Autodesk Inventor part; units mm, degrees
(part 2 of 2)
sketch "Boceto13" plane through (0, 0, 0) normal (0, 0, -1) x (-1, 0, 0)
  circle A0 centre (-56.75, 72.0206) radius 8 projected
  line L0 (-56.75, 72.0206) -> (-80.75, 72.0206)
  line L1 (-80.75, 105.95) -> (-80.75, -105.95) projected
  line L2 (-80.75, 72.0206) -> (80.75, 72.0206)
  line L3 (80.75, -105.95) -> (80.75, 105.95) projected
  circle A1 centre (-56.75, 43.1636) radius 8 projected
  line L4 (-56.75, 43.1636) -> (-56.75, 72.0206)
  line L5 (-56.75, 43.1636) -> (-80.75, 43.1636)
  line L6 (-80.75, 43.1636) -> (80.75, 43.1636)
  line L7 (-56.75, 14.3066) -> (-56.75, 43.1636)
  line L8 (-56.75, 14.3066) -> (-80.75, 14.3066)
  line L9 (-80.75, 14.3066) -> (80.75, 14.3066)
  line L10 (-56.75, -14.5504) -> (-56.75, 14.3066)
  line L11 (-56.75, -14.5504) -> (-80.75, -14.5504)
  line L12 (-80.75, -14.5504) -> (80.75, -14.5504)
  line L13 (-56.75, -43.4074) -> (-56.75, -14.5504)
  line L14 (-56.75, -43.4074) -> (-80.75, -43.4074)
  line L15 (-80.75, -43.4074) -> (80.75, -43.4074)
  line L16 (-56.75, -72.2644) -> (-56.75, -43.4074)
  line L17 (-56.75, -98.6167) -> (-56.75, -69.7597)
  line L18 (-56.75, -72.2644) -> (-80.75, -72.2644)
  line L19 (-80.75, -72.2644) -> (80.75, -72.2644)
  line L20 (-56.75, -101.1214) -> (-56.75, -72.2644)
  line L21 (43.5, 62.1456) -> (30.5, 62.1456) projected
  line L22 (30.5, 62.1456) -> (-80.75, 62.1456)
  line L23 (30.5, 81.8956) -> (43.5, 81.8956) projected
  line L24 (30.5, 81.8956) -> (80.75, 81.8956)
  line L25 (30.5, 62.1456) -> (80.75, 62.1456)
  line L26 (30.5, 81.8956) -> (-80.75, 81.8956)
  line L27 (30.5, 33.2886) -> (-80.75, 33.2886)
  line L28 (30.5, 53.0386) -> (80.75, 53.0386)
  line L29 (30.5, 33.2886) -> (80.75, 33.2886)
  line L30 (30.5, 53.0386) -> (-80.75, 53.0386)
  line L31 (30.5, 4.4316) -> (-80.75, 4.4316)
  line L32 (30.5, 24.1816) -> (80.75, 24.1816)
  line L33 (30.5, 4.4316) -> (80.75, 4.4316)
  line L34 (30.5, 24.1816) -> (-80.75, 24.1816)
  line L35 (30.5, -24.4254) -> (-80.75, -24.4254)
  line L36 (30.5, -4.6754) -> (80.75, -4.6754)
  line L37 (30.5, -24.4254) -> (80.75, -24.4254)
  line L38 (30.5, -4.6754) -> (-80.75, -4.6754)
  line L39 (30.5, -53.2824) -> (-80.75, -53.2824)
  line L40 (30.5, -33.5324) -> (80.75, -33.5324)
  line L41 (30.5, -53.2824) -> (80.75, -53.2824)
  line L42 (30.5, -33.5324) -> (-80.75, -33.5324)
  line L43 (30.5, -82.1394) -> (-80.75, -82.1394)
  line L44 (30.5, -62.3894) -> (80.75, -62.3894)
  line L45 (30.5, -82.1394) -> (80.75, -82.1394)
  line L46 (30.5, -62.3894) -> (-80.75, -62.3894)
  line L47 (-80.6263, 81.8524) -> (-64.7122, 81.8524) construction
  line L48 (-64.7122, 81.8524) -> (-64.7122, 62.1807) construction
  line L49 (-64.7122, 62.1807) -> (-80.6263, 62.1807) construction
  line L50 (-80.6263, 62.1807) -> (-80.6263, 81.8524) construction
  line L51 (-83, 108.2) -> (83, 108.2) projected
  line L52 (0, 108.2) -> (0, -109.1206)
  line L53 (-80.6263, 52.9954) -> (-64.7122, 52.9954) construction
  line L54 (-64.7122, 52.9954) -> (-64.7122, 33.3237) construction
  line L55 (-64.7122, 33.3237) -> (-80.6263, 33.3237) construction
  line L56 (-80.6263, 33.3237) -> (-80.6263, 52.9954) construction
  line L57 (-80.6263, 24.1384) -> (-64.7122, 24.1384) construction
  line L58 (-64.7122, 24.1384) -> (-64.7122, 4.4667) construction
  line L59 (-64.7122, 4.4667) -> (-80.6263, 4.4667) construction
  line L60 (-80.6263, 4.4667) -> (-80.6263, 24.1384) construction
  line L61 (-80.6263, -4.7186) -> (-64.7122, -4.7186) construction
  line L62 (-64.7122, -4.7186) -> (-64.7122, -24.3903) construction
  line L63 (-64.7122, -24.3903) -> (-80.6263, -24.3903) construction
  line L64 (-80.6263, -24.3903) -> (-80.6263, -4.7186) construction
  line L65 (-80.6263, -33.5756) -> (-64.7122, -33.5756) construction
  line L66 (-64.7122, -33.5756) -> (-64.7122, -53.2473) construction
  line L67 (-64.7122, -53.2473) -> (-80.6263, -53.2473) construction
  line L68 (-80.6263, -53.2473) -> (-80.6263, -33.5756) construction
  line L69 (-80.6263, -62.4326) -> (-64.7122, -62.4326) construction
  line L70 (-64.7122, -62.4326) -> (-64.7122, -82.1043) construction
  line L71 (-64.7122, -82.1043) -> (-80.6263, -82.1043) construction
  line L72 (-80.6263, -82.1043) -> (-80.6263, -62.4326) construction
  line L73 (-72.6693, 72.0206) -> (-88.5883, 72.0206)
  circle A2 centre (56.75, 72.0206) radius 8 projected
  circle A3 centre (56.75, -72.2644) radius 8 projected
  line L74 (56.75, 72.0206) -> (56.75, -72.2644)
  line L75 (64.7119, 81.8524) -> (80.6261, 81.8524) construction
  line L76 (80.6261, 81.8524) -> (80.6261, 62.1807) construction
  line L77 (80.6261, 62.1807) -> (64.7119, 62.1807) construction
  line L78 (64.7119, 62.1807) -> (64.7119, 81.8524) construction
  line L79 (56.75, 43.1636) -> (56.75, 14.3066)
  line L80 (56.75, -14.5504) -> (56.75, 14.3066)
  circle A4 centre (56.75, -43.4074) radius 8 projected
  line L81 (56.75, -72.2644) -> (56.75, -43.4074)
  line L82 (56.75, -43.4074) -> (56.75, -14.5504)
  line L83 (64.7119, 33.3237) -> (64.7119, 52.9954) construction
  line L84 (64.7119, 52.9954) -> (80.6261, 52.9954) construction
  line L85 (80.6261, 52.9954) -> (80.6261, 33.3237) construction
  line L86 (80.6261, 33.3237) -> (64.7119, 33.3237) construction
  line L87 (64.7119, 4.4667) -> (64.7119, 24.1384) construction
  line L88 (64.7119, 24.1384) -> (80.6261, 24.1384) construction
  line L89 (80.6261, 24.1384) -> (80.6261, 4.4667) construction
  line L90 (80.6261, 4.4667) -> (64.7119, 4.4667) construction
  line L91 (64.7119, -24.3903) -> (64.7119, -4.7186) construction
  line L92 (64.7119, -4.7186) -> (80.6261, -4.7186) construction
  line L93 (80.6261, -4.7186) -> (80.6261, -24.3903) construction
  line L94 (80.6261, -24.3903) -> (64.7119, -24.3903) construction
  line L95 (64.7119, -53.2473) -> (64.7119, -33.5756) construction
  line L96 (64.7119, -33.5756) -> (80.6261, -33.5756) construction
  line L97 (80.6261, -33.5756) -> (80.6261, -53.2473) construction
  line L98 (80.6261, -53.2473) -> (64.7119, -53.2473) construction
  line L99 (64.7119, -82.1043) -> (64.7119, -62.4326) construction
  line L100 (64.7119, -62.4326) -> (80.6261, -62.4326) construction
  line L101 (80.6261, -62.4326) -> (80.6261, -82.1043) construction
  line L102 (80.6261, -82.1043) -> (64.7119, -82.1043) construction
  line L103 (-70.5115, 68.9591) -> (-74.5403, 68.9591)
  line L104 (-74.5403, 68.9591) -> (-74.5403, 70.0219)
  line L105 (-74.5403, 70.0219) -> (-73.2551, 70.0219)
  line L106 (-73.2551, 70.0219) -> (-73.2551, 73.2499)
  line L107 (-73.2551, 73.2499) -> (-74.5403, 73.2499)
  line L108 (-74.5403, 73.2499) -> (-74.5403, 74.2435)
  spline S0 degree 2 poles (-74.5403, 74.2435) (-74.2585, 74.2435) (-73.7, 74.3177) (-73.5319, 74.3967) knots 0 0 0 1 2 2 2
  spline S1 degree 2 poles (-73.5319, 74.3967) (-73.3391, 74.4956) (-73.1216, 74.8268) (-73.1018, 75.074) knots 0 0 0 1 2 2 2
  line L109 (-73.1018, 75.074) -> (-71.7671, 75.074)
  line L110 (-71.7671, 75.074) -> (-71.7671, 70.0219)
  line L111 (-71.7671, 70.0219) -> (-70.5115, 70.0219)
  line L112 (-70.5115, 70.0219) -> (-70.5115, 68.9591)
  line L113 (-70.2397, 40.0502) -> (-74.7232, 40.0502)
  line L114 (-74.7232, 40.0502) -> (-74.7232, 41.0438)
  spline S2 degree 2 poles (-74.7232, 41.0438) (-74.1547, 41.4986) (-73.2452, 42.2994) (-72.9041, 42.6603) knots 0 0 0 1 2 2 2
  spline S3 degree 2 poles (-72.9041, 42.6603) (-72.4542, 43.1299) (-72.0538, 43.8467) (-72.0538, 44.2224) knots 0 0 0 1 2 2 2
  spline S4 degree 2 poles (-72.0538, 44.2224) (-72.0538, 44.6475) (-72.563, 45.1023) (-73.0178, 45.1023) knots 0 0 0 1 2 2 2
  spline S5 degree 2 poles (-73.0178, 45.1023) (-73.2501, 45.1023) (-73.6653, 44.9886) (-73.8779, 44.8996) knots 0 0 0 1 2 2 2
  spline S6 degree 2 poles (-73.8779, 44.8996) (-74.0855, 44.8057) (-74.3821, 44.6079) (-74.4563, 44.5585) knots 0 0 0 1 2 2 2
  line L115 (-74.4563, 44.5585) -> (-74.5749, 44.5585)
  line L116 (-74.5749, 44.5585) -> (-74.5749, 45.8882)
  spline S7 degree 2 poles (-74.5749, 45.8882) (-74.3179, 46.0118) (-73.2205, 46.2689) (-72.7113, 46.2689) knots 0 0 0 1 2 2 2
  spline S8 degree 2 poles (-72.7113, 46.2689) (-71.6238, 46.2689) (-70.5066, 45.3) (-70.5066, 44.425) knots 0 0 0 1 2 2 2
  spline S9 degree 2 poles (-70.5066, 44.425) (-70.5066, 43.8862) (-71.0158, 42.8481) (-71.604, 42.2549) knots 0 0 0 1 2 2 2
  spline S10 degree 2 poles (-71.604, 42.2549) (-71.9748, 41.8891) (-72.6718, 41.3207) (-72.825, 41.202) knots 0 0 0 1 2 2 2
  line L117 (-72.825, 41.202) -> (-70.2397, 41.202)
  line L118 (-70.2397, 41.202) -> (-70.2397, 40.0502)
  spline S11 degree 2 poles (-70.3929, 13.1013) (-70.3929, 12.6515) (-70.7241, 11.915) (-71.0454, 11.6579) knots 0 0 0 1 2 2 2
  spline S12 degree 2 poles (-71.0454, 11.6579) (-71.3667, 11.4009) (-72.2417, 11.124) (-72.8695, 11.124) knots 0 0 0 1 2 2 2
  spline S13 degree 2 poles (-72.8695, 11.124) (-73.5813, 11.124) (-74.5996, 11.3613) (-74.9209, 11.5096) knots 0 0 0 1 2 2 2
  line L119 (-74.9209, 11.5096) -> (-74.9209, 12.8344)
  line L120 (-74.9209, 12.8344) -> (-74.7726, 12.8344)
  spline S14 degree 2 poles (-74.7726, 12.8344) (-74.4365, 12.6218) (-73.5319, 12.3055) (-73.1562, 12.3055) knots 0 0 0 1 2 2 2
  spline S15 degree 2 poles (-73.1562, 12.3055) (-72.9337, 12.3055) (-72.4147, 12.3846) (-72.2367, 12.5131) knots 0 0 0 1 2 2 2
  spline S16 degree 2 poles (-72.2367, 12.5131) (-72.0983, 12.6169) (-71.9303, 12.9184) (-71.9303, 13.1903) knots 0 0 0 1 2 2 2
  spline S17 degree 2 poles (-71.9303, 13.1903) (-71.9303, 13.4622) (-72.1675, 13.7539) (-72.3653, 13.8231) knots 0 0 0 1 2 2 2
  spline S18 degree 2 poles (-72.3653, 13.8231) (-72.563, 13.8923) (-73.1117, 13.9071) (-73.3243, 13.9071) knots 0 0 0 1 2 2 2
  line L121 (-73.3243, 13.9071) -> (-73.5863, 13.9071)
  line L122 (-73.5863, 13.9071) -> (-73.5863, 14.9798)
  line L123 (-73.5863, 14.9798) -> (-73.344, 14.9798)
  spline S19 degree 2 poles (-73.344, 14.9798) (-73.0672, 14.9798) (-72.5976, 15.0292) (-72.4345, 15.1034) knots 0 0 0 1 2 2 2
  spline S20 degree 2 poles (-72.4345, 15.1034) (-72.2713, 15.1825) (-72.0884, 15.4593) (-72.0884, 15.6966) knots 0 0 0 1 2 2 2
  spline S21 degree 2 poles (-72.0884, 15.6966) (-72.0884, 15.8844) (-72.2615, 16.1167) (-72.385, 16.181) knots 0 0 0 1 2 2 2
  spline S22 degree 2 poles (-72.385, 16.181) (-72.5333, 16.2551) (-72.9288, 16.3046) (-73.0672, 16.3046) knots 0 0 0 1 2 2 2
  spline S23 degree 2 poles (-73.0672, 16.3046) (-73.2897, 16.3046) (-73.7593, 16.2008) (-73.9768, 16.1167) knots 0 0 0 1 2 2 2
  spline S24 degree 2 poles (-73.9768, 16.1167) (-74.1498, 16.0525) (-74.5255, 15.8449) (-74.6145, 15.7905) knots 0 0 0 1 2 2 2
  line L124 (-74.6145, 15.7905) -> (-74.743, 15.7905)
  line L125 (-74.743, 15.7905) -> (-74.743, 17.0955)
  spline S25 degree 2 poles (-74.743, 17.0955) (-74.4266, 17.229) (-73.3589, 17.4811) (-72.8003, 17.4811) knots 0 0 0 1 2 2 2
  spline S26 degree 2 poles (-72.8003, 17.4811) (-72.2565, 17.4811) (-71.4557, 17.2932) (-71.1739, 17.1103) knots 0 0 0 1 2 2 2
  spline S27 degree 2 poles (-71.1739, 17.1103) (-70.8625, 16.9175) (-70.5511, 16.3244) (-70.5511, 15.9536) knots 0 0 0 1 2 2 2
  spline S28 degree 2 poles (-70.5511, 15.9536) (-70.5511, 15.4296) (-71.1542, 14.6486) (-71.6485, 14.5349) knots 0 0 0 1 2 2 2
  line L126 (-71.6485, 14.5349) -> (-71.6485, 14.4756)
  spline S29 degree 2 poles (-71.6485, 14.4756) (-71.431, 14.4459) (-71.0158, 14.2877) (-70.818, 14.1098) knots 0 0 0 1 2 2 2
  spline S30 degree 2 poles (-70.818, 14.1098) (-70.6351, 13.9516) (-70.3929, 13.4474) (-70.3929, 13.1013) knots 0 0 0 1 2 2 2
  line L127 (-70.1655, -16.1734) -> (-70.991, -16.1734)
  line L128 (-70.991, -16.1734) -> (-70.991, -17.6119)
  line L129 (-70.991, -17.6119) -> (-72.4691, -17.6119)
  line L130 (-72.4691, -17.6119) -> (-72.4691, -16.1734)
  line L131 (-72.4691, -16.1734) -> (-75.1582, -16.1734)
  line L132 (-75.1582, -16.1734) -> (-75.1582, -15.0364)
  line L133 (-75.1582, -15.0364) -> (-72.5185, -11.497)
  line L134 (-72.5185, -11.497) -> (-70.991, -11.497)
  line L135 (-70.991, -11.497) -> (-70.991, -15.076)
  line L136 (-70.991, -15.076) -> (-70.1655, -15.076)
  line L137 (-70.1655, -15.076) -> (-70.1655, -16.1734)
  line L138 (-72.4691, -15.076) -> (-72.4691, -12.9998)
  line L139 (-72.4691, -12.9998) -> (-74.0163, -15.076)
  line L140 (-74.0163, -15.076) -> (-72.4691, -15.076)
  spline S31 degree 2 poles (-70.3781, -44.3309) (-70.3781, -44.8104) (-70.7043, -45.6211) (-71.0256, -45.9127) knots 0 0 0 1 2 2 2
  spline S32 degree 2 poles (-71.0256, -45.9127) (-71.347, -46.2044) (-72.2269, -46.5257) (-72.8695, -46.5257) knots 0 0 0 1 2 2 2
  spline S33 degree 2 poles (-72.8695, -46.5257) (-73.5517, -46.5208) (-74.5304, -46.2983) (-74.8517, -46.155) knots 0 0 0 1 2 2 2
  line L141 (-74.8517, -46.155) -> (-74.8517, -44.8252)
  line L142 (-74.8517, -44.8252) -> (-74.7133, -44.8252)
  spline S34 degree 2 poles (-74.7133, -44.8252) (-74.5947, -44.8895) (-74.308, -45.0576) (-74.0756, -45.1465) knots 0 0 0 1 2 2 2
  spline S35 degree 2 poles (-74.0756, -45.1465) (-73.8581, -45.2306) (-73.4083, -45.3443) (-73.1364, -45.3443) knots 0 0 0 1 2 2 2
  spline S36 degree 2 poles (-73.1364, -45.3443) (-72.8991, -45.3443) (-72.3455, -45.2256) (-72.1774, -45.0674) knots 0 0 0 1 2 2 2
  spline S37 degree 2 poles (-72.1774, -45.0674) (-72.0538, -44.9439) (-71.9154, -44.6423) (-71.9154, -44.3902) knots 0 0 0 1 2 2 2
  spline S38 degree 2 poles (-71.9154, -44.3902) (-71.9154, -44.1727) (-72.0934, -43.8662) (-72.2367, -43.7723) knots 0 0 0 1 2 2 2
  spline S39 degree 2 poles (-72.2367, -43.7723) (-72.4444, -43.6339) (-73.0376, -43.5548) (-73.2501, -43.5548) knots 0 0 0 1 2 2 2
  spline S40 degree 2 poles (-73.2501, -43.5548) (-73.5863, -43.5548) (-74.2239, -43.6636) (-74.4563, -43.7229) knots 0 0 0 1 2 2 2
  line L143 (-74.4563, -43.7229) -> (-74.5897, -43.7229)
  line L144 (-74.5897, -43.7229) -> (-74.5897, -40.2972)
  line L145 (-74.5897, -40.2972) -> (-70.5461, -40.2972)
  line L146 (-70.5461, -40.2972) -> (-70.5461, -41.449)
  line L147 (-70.5461, -41.449) -> (-73.1414, -41.449)
  line L148 (-73.1414, -41.449) -> (-73.1414, -42.4623)
  spline S41 degree 2 poles (-73.1414, -42.4623) (-73.0178, -42.4524) (-72.6767, -42.4426) (-72.5828, -42.4426) knots 0 0 0 1 2 2 2
  spline S42 degree 2 poles (-72.5828, -42.4426) (-72.1428, -42.4426) (-71.4013, -42.6205) (-71.1097, -42.8034) knots 0 0 0 1 2 2 2
  spline S43 degree 2 poles (-71.1097, -42.8034) (-70.7636, -43.0308) (-70.3781, -43.7871) (-70.3781, -44.3309) knots 0 0 0 1 2 2 2
  spline S44 degree 2 poles (-70.2743, -73.2349) (-70.2743, -74.1988) (-71.4953, -75.4396) (-72.563, -75.4396) knots 0 0 0 1 2 2 2
  spline S45 degree 2 poles (-72.563, -75.4396) (-73.0969, -75.4396) (-73.9323, -75.1331) (-74.2239, -74.8315) knots 0 0 0 1 2 2 2
  spline S46 degree 2 poles (-74.2239, -74.8315) (-74.57, -74.4806) (-74.9407, -73.3683) (-74.9407, -72.5922) knots 0 0 0 1 2 2 2
  spline S47 degree 2 poles (-74.9407, -72.5922) (-74.9407, -71.7914) (-74.5947, -70.5457) (-74.2042, -70.0662) knots 0 0 0 1 2 2 2
  spline S48 degree 2 poles (-74.2042, -70.0662) (-73.8334, -69.6114) (-72.6273, -69.0973) (-71.8017, -69.0973) knots 0 0 0 1 2 2 2
  spline S49 degree 2 poles (-71.8017, -69.0973) (-71.5002, -69.0973) (-70.8971, -69.1764) (-70.7884, -69.2011) knots 0 0 0 1 2 2 2
  line L149 (-70.7884, -69.2011) -> (-70.7884, -70.3974)
  line L150 (-70.7884, -70.3974) -> (-70.8971, -70.3974)
  spline S50 degree 2 poles (-70.8971, -70.3974) (-71.0059, -70.343) (-71.5002, -70.2096) (-71.8166, -70.2096) knots 0 0 0 1 2 2 2
  spline S51 degree 2 poles (-71.8166, -70.2096) (-72.5333, -70.2096) (-73.3144, -70.9659) (-73.4083, -71.6678) knots 0 0 0 1 2 2 2
  spline S52 degree 2 poles (-73.4083, -71.6678) (-73.1068, -71.475) (-72.4889, -71.2477) (-72.0983, -71.2477) knots 0 0 0 1 2 2 2
  spline S53 degree 2 poles (-72.0983, -71.2477) (-71.7671, -71.2477) (-71.1888, -71.4256) (-70.9663, -71.5937) knots 0 0 0 1 2 2 2
  spline S54 degree 2 poles (-70.9663, -71.5937) (-70.65, -71.8359) (-70.2743, -72.6219) (-70.2743, -73.2349) knots 0 0 0 1 2 2 2
  spline S55 degree 2 poles (-72.0588, -74.1543) (-71.9401, -74.006) (-71.8116, -73.66) (-71.8116, -73.309) knots 0 0 0 1 2 2 2
  spline S56 degree 2 poles (-71.8116, -73.309) (-71.8116, -73.0124) (-71.9599, -72.6268) (-72.0934, -72.5131) knots 0 0 0 1 2 2 2
  spline S57 degree 2 poles (-72.0934, -72.5131) (-72.2318, -72.3945) (-72.5729, -72.3105) (-72.7657, -72.3105) knots 0 0 0 1 2 2 2
  spline S58 degree 2 poles (-72.7657, -72.3105) (-72.9288, -72.3105) (-73.2649, -72.3945) (-73.4132, -72.4538) knots 0 0 0 1 2 2 2
  spline S59 degree 2 poles (-73.4132, -72.4538) (-73.4132, -72.4934) (-73.4231, -72.6812) (-73.4231, -72.8246) knots 0 0 0 1 2 2 2
  spline S60 degree 2 poles (-73.4231, -72.8246) (-73.4231, -73.3535) (-73.2402, -73.9912) (-73.0969, -74.1543) knots 0 0 0 1 2 2 2
  spline S61 degree 2 poles (-73.0969, -74.1543) (-72.9931, -74.2878) (-72.7162, -74.4015) (-72.5679, -74.4015) knots 0 0 0 1 2 2 2
  spline S62 degree 2 poles (-72.5679, -74.4015) (-72.4444, -74.4015) (-72.1577, -74.2779) (-72.0588, -74.1543) knots 0 0 0 1 2 2 2
  line L151 (74.9652, 73.8555) -> (72.36, 68.9666)
  line L152 (72.36, 68.9666) -> (70.6596, 68.9666)
  line L153 (70.6596, 68.9666) -> (73.3833, 73.9148)
  line L154 (73.3833, 73.9148) -> (70.4767, 73.9148)
  line L155 (70.4767, 73.9148) -> (70.4767, 75.0666)
  line L156 (70.4767, 75.0666) -> (74.9652, 75.0666)
  line L157 (74.9652, 75.0666) -> (74.9652, 73.8555)
  spline S63 degree 2 poles (75.0838, 41.8076) (75.0838, 41.4171) (74.7575, 40.7398) (74.4461, 40.4927) knots 0 0 0 1 2 2 2
  spline S64 degree 2 poles (74.4461, 40.4927) (74.1347, 40.2455) (73.2399, 39.9687) (72.6616, 39.9687) knots 0 0 0 1 2 2 2
  spline S65 degree 2 poles (72.6616, 39.9687) (72.0437, 39.9687) (71.1193, 40.2504) (70.8227, 40.4927) knots 0 0 0 1 2 2 2
  spline S66 degree 2 poles (70.8227, 40.4927) (70.531, 40.7349) (70.2542, 41.3923) (70.2542, 41.7581) knots 0 0 0 1 2 2 2
  spline S67 degree 2 poles (70.2542, 41.7581) (70.2542, 42.2821) (70.8326, 42.9791) (71.3813, 43.2115) knots 0 0 0 1 2 2 2
  line L158 (71.3813, 43.2115) -> (71.3813, 43.2362)
  spline S68 degree 2 poles (71.3813, 43.2362) (70.8425, 43.4982) (70.4173, 44.2446) (70.4173, 44.7043) knots 0 0 0 1 2 2 2
  spline S69 degree 2 poles (70.4173, 44.7043) (70.4173, 45.0405) (70.7139, 45.6287) (71.0056, 45.8611) knots 0 0 0 1 2 2 2
  spline S70 degree 2 poles (71.0056, 45.8611) (71.2874, 46.0835) (72.1425, 46.3504) (72.6764, 46.3504) knots 0 0 0 1 2 2 2
  spline S71 degree 2 poles (72.6764, 46.3504) (73.2399, 46.3504) (74.0803, 46.1082) (74.3522, 45.9105) knots 0 0 0 1 2 2 2
  spline S72 degree 2 poles (74.3522, 45.9105) (74.629, 45.7128) (74.9256, 45.1393) (74.9256, 44.8081) knots 0 0 0 1 2 2 2
  spline S73 degree 2 poles (74.9256, 44.8081) (74.9256, 44.3731) (74.4214, 43.6761) (73.9023, 43.4339) knots 0 0 0 1 2 2 2
  line L159 (73.9023, 43.4339) -> (73.9023, 43.4141)
  spline S74 degree 2 poles (73.9023, 43.4141) (74.5104, 43.167) (75.0838, 42.3662) (75.0838, 41.8076) knots 0 0 0 1 2 2 2
  spline S75 degree 2 poles (73.5711, 41.7433) (73.5711, 42.0448) (73.3141, 42.3612) (72.8989, 42.5639) knots 0 0 0 1 2 2 2
  spline S76 degree 2 poles (72.8989, 42.5639) (72.7802, 42.6183) (72.3304, 42.7913) (72.1574, 42.8654) knots 0 0 0 1 2 2 2
  spline S77 degree 2 poles (72.1574, 42.8654) (71.9992, 42.7072) (71.7471, 42.2327) (71.7471, 41.9509) knots 0 0 0 1 2 2 2
  spline S78 degree 2 poles (71.7471, 41.9509) (71.7471, 41.5258) (72.2908, 41.0166) (72.7308, 41.0166) knots 0 0 0 1 2 2 2
  spline S79 degree 2 poles (72.7308, 41.0166) (72.8544, 41.0166) (73.1609, 41.0957) (73.2795, 41.1748) knots 0 0 0 1 2 2 2
  spline S80 degree 2 poles (73.2795, 41.1748) (73.413, 41.2688) (73.5711, 41.5258) (73.5711, 41.7433) knots 0 0 0 1 2 2 2
  spline S81 degree 2 poles (73.4377, 44.6302) (73.4377, 44.9416) (73.0274, 45.3124) (72.6764, 45.3124) knots 0 0 0 1 2 2 2
  spline S82 degree 2 poles (72.6764, 45.3124) (72.3403, 45.3124) (71.93, 44.9762) (71.93, 44.729) knots 0 0 0 1 2 2 2
  spline S83 degree 2 poles (71.93, 44.729) (71.93, 44.4868) (72.1771, 44.1853) (72.4391, 44.0617) knots 0 0 0 1 2 2 2
  spline S84 degree 2 poles (72.4391, 44.0617) (72.5528, 44.0024) (72.8692, 43.8788) (73.1312, 43.7799) knots 0 0 0 1 2 2 2
  spline S85 degree 2 poles (73.1312, 43.7799) (73.2894, 43.9876) (73.4377, 44.3781) (73.4377, 44.6302) knots 0 0 0 1 2 2 2
  spline S86 degree 2 poles (74.9404, 14.6412) (74.9404, 13.8651) (74.5796, 12.5699) (74.1989, 12.1053) knots 0 0 0 1 2 2 2
  spline S87 degree 2 poles (74.1989, 12.1053) (73.8035, 11.6357) (72.6369, 11.1314) (71.7866, 11.1314) knots 0 0 0 1 2 2 2
  spline S88 degree 2 poles (71.7866, 11.1314) (71.4999, 11.1314) (70.8771, 11.2056) (70.7733, 11.2353) knots 0 0 0 1 2 2 2
  line L160 (70.7733, 11.2353) -> (70.7733, 12.4315)
  line L161 (70.7733, 12.4315) -> (70.8919, 12.4315)
  spline S89 degree 2 poles (70.8919, 12.4315) (71.0056, 12.3722) (71.4307, 12.2437) (71.8015, 12.2437) knots 0 0 0 1 2 2 2
  spline S90 degree 2 poles (71.8015, 12.2437) (72.103, 12.2437) (72.6616, 12.4019) (72.8593, 12.5749) knots 0 0 0 1 2 2 2
  spline S91 degree 2 poles (72.8593, 12.5749) (73.0719, 12.7578) (73.3487, 13.2966) (73.3981, 13.7019) knots 0 0 0 1 2 2 2
  spline S92 degree 2 poles (73.3981, 13.7019) (73.0719, 13.4993) (72.5083, 13.2818) (72.0882, 13.2818) knots 0 0 0 1 2 2 2
  spline S93 degree 2 poles (72.0882, 13.2818) (71.7767, 13.2818) (71.1984, 13.4498) (70.9611, 13.6278) knots 0 0 0 1 2 2 2
  spline S94 degree 2 poles (70.9611, 13.6278) (70.6447, 13.87) (70.274, 14.6461) (70.274, 15.2591) knots 0 0 0 1 2 2 2
  spline S95 degree 2 poles (70.274, 15.2591) (70.274, 15.7386) (70.6002, 16.5443) (70.8968, 16.8409) knots 0 0 0 1 2 2 2
  spline S96 degree 2 poles (70.8968, 16.8409) (71.1934, 17.1375) (72.0536, 17.4737) (72.5825, 17.4737) knots 0 0 0 1 2 2 2
  spline S97 degree 2 poles (72.5825, 17.4737) (73.1164, 17.4737) (73.9419, 17.1771) (74.2385, 16.8656) knots 0 0 0 1 2 2 2
  spline S98 degree 2 poles (74.2385, 16.8656) (74.5845, 16.5196) (74.9404, 15.4222) (74.9404, 14.6412) knots 0 0 0 1 2 2 2
  spline S99 degree 2 poles (73.4228, 14.8686) (73.4228, 15.3678) (73.2548, 16.0105) (73.1015, 16.1884) knots 0 0 0 1 2 2 2
  spline S100 degree 2 poles (73.1015, 16.1884) (72.9977, 16.3219) (72.7308, 16.4356) (72.5775, 16.4356) knots 0 0 0 1 2 2 2
  spline S101 degree 2 poles (72.5775, 16.4356) (72.4391, 16.4356) (72.1821, 16.3268) (72.0634, 16.1884) knots 0 0 0 1 2 2 2
  spline S102 degree 2 poles (72.0634, 16.1884) (71.9596, 16.0698) (71.8113, 15.6101) (71.8113, 15.3382) knots 0 0 0 1 2 2 2
  spline S103 degree 2 poles (71.8113, 15.3382) (71.8113, 15.0416) (71.9646, 14.6609) (72.0931, 14.5472) knots 0 0 0 1 2 2 2
  spline S104 degree 2 poles (72.0931, 14.5472) (72.2266, 14.4336) (72.5578, 14.3446) (72.7654, 14.3446) knots 0 0 0 1 2 2 2
  spline S105 degree 2 poles (72.7654, 14.3446) (72.9384, 14.3446) (73.2993, 14.4385) (73.413, 14.4879) knots 0 0 0 1 2 2 2
  spline S106 degree 2 poles (73.413, 14.4879) (73.413, 14.5324) (73.4228, 14.7005) (73.4228, 14.8686) knots 0 0 0 1 2 2 2
  line L162 (72.1549, -17.602) -> (68.1261, -17.602)
  line L163 (68.1261, -17.602) -> (68.1261, -16.5392)
  line L164 (68.1261, -16.5392) -> (69.4114, -16.5392)
  line L165 (69.4114, -16.5392) -> (69.4114, -13.3112)
  line L166 (69.4114, -13.3112) -> (68.1261, -13.3112)
  line L167 (68.1261, -13.3112) -> (68.1261, -12.3176)
  spline S107 degree 2 poles (68.1261, -12.3176) (68.4079, -12.3176) (68.9665, -12.2435) (69.1346, -12.1644) knots 0 0 0 1 2 2 2
  spline S108 degree 2 poles (69.1346, -12.1644) (69.3273, -12.0655) (69.5449, -11.7343) (69.5646, -11.4871) knots 0 0 0 1 2 2 2
  line L168 (69.5646, -11.4871) -> (70.8993, -11.4871)
  line L169 (70.8993, -11.4871) -> (70.8993, -16.5392)
  line L170 (70.8993, -16.5392) -> (72.1549, -16.5392)
  line L171 (72.1549, -16.5392) -> (72.1549, -17.602)
  spline S109 degree 2 poles (77.6914, -14.552) (77.6914, -15.3429) (77.4393, -16.5293) (77.1575, -16.9297) knots 0 0 0 1 2 2 2
  spline S110 degree 2 poles (77.1575, -16.9297) (76.8807, -17.3251) (75.9859, -17.7305) (75.3433, -17.7305) knots 0 0 0 1 2 2 2
  spline S111 degree 2 poles (75.3433, -17.7305) (74.6957, -17.7305) (73.806, -17.3251) (73.5242, -16.9198) knots 0 0 0 1 2 2 2
  spline S112 degree 2 poles (73.5242, -16.9198) (73.2424, -16.5194) (72.9903, -15.3429) (72.9903, -14.552) knots 0 0 0 1 2 2 2
  spline S113 degree 2 poles (72.9903, -14.552) (72.9903, -13.7413) (73.2424, -12.5944) (73.5291, -12.1792) knots 0 0 0 1 2 2 2
  spline S114 degree 2 poles (73.5291, -12.1792) (73.8158, -11.7739) (74.7205, -11.3784) (75.3433, -11.3784) knots 0 0 0 1 2 2 2
  spline S115 degree 2 poles (75.3433, -11.3784) (76.0008, -11.3784) (76.8807, -11.7936) (77.1624, -12.2039) knots 0 0 0 1 2 2 2
  spline S116 degree 2 poles (77.1624, -12.2039) (77.4393, -12.6043) (77.6914, -13.7858) (77.6914, -14.552) knots 0 0 0 1 2 2 2
  spline S117 degree 2 poles (76.154, -14.552) (76.154, -13.42) (75.7833, -12.5055) (75.3433, -12.5055) knots 0 0 0 1 2 2 2
  spline S118 degree 2 poles (75.3433, -12.5055) (74.9034, -12.5055) (74.5277, -13.42) (74.5277, -14.5569) knots 0 0 0 1 2 2 2
  spline S119 degree 2 poles (74.5277, -14.5569) (74.5277, -15.6741) (74.9034, -16.6034) (75.3433, -16.6034) knots 0 0 0 1 2 2 2
  spline S120 degree 2 poles (75.3433, -16.6034) (75.7783, -16.6034) (76.154, -15.6741) (76.154, -14.552) knots 0 0 0 1 2 2 2
  line L172 (72.1549, -46.4689) -> (68.1261, -46.4689)
  line L173 (68.1261, -46.4689) -> (68.1261, -45.4061)
  line L174 (68.1261, -45.4061) -> (69.4114, -45.4061)
  line L175 (69.4114, -45.4061) -> (69.4114, -42.1781)
  line L176 (69.4114, -42.1781) -> (68.1261, -42.1781)
  line L177 (68.1261, -42.1781) -> (68.1261, -41.1845)
  spline S121 degree 2 poles (68.1261, -41.1845) (68.4079, -41.1845) (68.9665, -41.1103) (69.1346, -41.0313) knots 0 0 0 1 2 2 2
  spline S122 degree 2 poles (69.1346, -41.0313) (69.3273, -40.9324) (69.5449, -40.6012) (69.5646, -40.354) knots 0 0 0 1 2 2 2
  line L178 (69.5646, -40.354) -> (70.8993, -40.354)
  line L179 (70.8993, -40.354) -> (70.8993, -45.4061)
  line L180 (70.8993, -45.4061) -> (72.1549, -45.4061)
  line L181 (72.1549, -45.4061) -> (72.1549, -46.4689)
  line L182 (77.4986, -46.4689) -> (73.4698, -46.4689)
  line L183 (73.4698, -46.4689) -> (73.4698, -45.4061)
  line L184 (73.4698, -45.4061) -> (74.7551, -45.4061)
  line L185 (74.7551, -45.4061) -> (74.7551, -42.1781)
  line L186 (74.7551, -42.1781) -> (73.4698, -42.1781)
  line L187 (73.4698, -42.1781) -> (73.4698, -41.1845)
  spline S123 degree 2 poles (73.4698, -41.1845) (73.7516, -41.1845) (74.3102, -41.1103) (74.4782, -41.0313) knots 0 0 0 1 2 2 2
  spline S124 degree 2 poles (74.4782, -41.0313) (74.671, -40.9324) (74.8885, -40.6012) (74.9083, -40.354) knots 0 0 0 1 2 2 2
  line L188 (74.9083, -40.354) -> (76.243, -40.354)
  line L189 (76.243, -40.354) -> (76.243, -45.4061)
  line L190 (76.243, -45.4061) -> (77.4986, -45.4061)
  line L191 (77.4986, -45.4061) -> (77.4986, -46.4689)
  line L192 (72.1549, -75.3778) -> (68.1261, -75.3778)
  line L193 (68.1261, -75.3778) -> (68.1261, -74.315)
  line L194 (68.1261, -74.315) -> (69.4114, -74.315)
  line L195 (69.4114, -74.315) -> (69.4114, -71.087)
  line L196 (69.4114, -71.087) -> (68.1261, -71.087)
  line L197 (68.1261, -71.087) -> (68.1261, -70.0934)
  spline S125 degree 2 poles (68.1261, -70.0934) (68.4079, -70.0934) (68.9665, -70.0193) (69.1346, -69.9402) knots 0 0 0 1 2 2 2
  spline S126 degree 2 poles (69.1346, -69.9402) (69.3273, -69.8413) (69.5449, -69.5101) (69.5646, -69.2629) knots 0 0 0 1 2 2 2
  line L198 (69.5646, -69.2629) -> (70.8993, -69.2629)
  line L199 (70.8993, -69.2629) -> (70.8993, -74.315)
  line L200 (70.8993, -74.315) -> (72.1549, -74.315)
  line L201 (72.1549, -74.315) -> (72.1549, -75.3778)
  line L202 (77.7705, -75.3778) -> (73.2869, -75.3778)
  line L203 (73.2869, -75.3778) -> (73.2869, -74.3842)
  spline S127 degree 2 poles (73.2869, -74.3842) (73.8554, -73.9294) (74.7649, -73.1286) (75.106, -72.7677) knots 0 0 0 1 2 2 2
  spline S128 degree 2 poles (75.106, -72.7677) (75.5559, -72.2981) (75.9563, -71.5813) (75.9563, -71.2056) knots 0 0 0 1 2 2 2
  spline S129 degree 2 poles (75.9563, -71.2056) (75.9563, -70.7805) (75.4471, -70.3257) (74.9923, -70.3257) knots 0 0 0 1 2 2 2
  spline S130 degree 2 poles (74.9923, -70.3257) (74.76, -70.3257) (74.3448, -70.4394) (74.1322, -70.5284) knots 0 0 0 1 2 2 2
  spline S131 degree 2 poles (74.1322, -70.5284) (73.9246, -70.6223) (73.628, -70.8201) (73.5538, -70.8695) knots 0 0 0 1 2 2 2
  line L204 (73.5538, -70.8695) -> (73.4352, -70.8695)
  line L205 (73.4352, -70.8695) -> (73.4352, -69.5398)
  spline S132 degree 2 poles (73.4352, -69.5398) (73.6923, -69.4162) (74.7897, -69.1591) (75.2988, -69.1591) knots 0 0 0 1 2 2 2
  spline S133 degree 2 poles (75.2988, -69.1591) (76.3863, -69.1591) (77.5035, -70.128) (77.5035, -71.003) knots 0 0 0 1 2 2 2
  spline S134 degree 2 poles (77.5035, -71.003) (77.5035, -71.5418) (76.9944, -72.5799) (76.4061, -73.1731) knots 0 0 0 1 2 2 2
  spline S135 degree 2 poles (76.4061, -73.1731) (76.0354, -73.5389) (75.3384, -74.1073) (75.1851, -74.226) knots 0 0 0 1 2 2 2
  line L206 (75.1851, -74.226) -> (77.7705, -74.226)
  line L207 (77.7705, -74.226) -> (77.7705, -75.3778)
  point P0 (0, 0)
  constraints: 100 end point, 20 point on line, 12 horizontal, 9 vertical, 3 collinear, 3 perpendicular, 1 midpoint, 24 other
extrude "Extrusión13" cut sketch "Boceto13" against normal blind 1.5 contours L110 L111 L112 L103 L104 L105 L106 L0 | L0 L106 L107 L108 S0 S1 L109 L110 | L153 L154 L155 L156 L157 L151 L2 | L2 L151 L152 L153 | S9 S10 L117 L118 L113 L114 S2 S3 L5 | L5 S3 S4 S5 S6 L115 L116 S7 S8 S9 | S67 L158 S68 S69 S70 S71 S72 S73 L159 S74 L6 | L6 S74 S63 S64 S65 S66 S67 | L122 L123 S19 S20 S21 S22 S23 S24 L124 L125 S25 S26 S27 S28 L126 S29 L8 | L8 S29 S30 S11 S12 S13 L119 L120 S14 S15 S16 S17 S18 L121 L122 | S94 S95 S96 S97 S98 S86 L9 | L9 S86 S87 S88 L160 L161 S89 S90 S91 S92 S93 S94 | L133 L134 L135 L11 L138 L139 | L11 L139 L140 L138 L135 L136 L137 L127 L128 L129 L130 L131 L132 L133 | L165 L166 L167 S107 S108 L168 L169 L12 | L12 L169 L170 L171 L162 L163 L164 L165 | S109 S110 S111 S112 L12 S118 S119 S120 | L12 S117 S118 S113 S114 S115 S116 | L144 L145 L146 L147 L148 S41 S42 S43 L14 | L14 S43 S31 S32 S33 L141 L142 S34 S35 S36 S37 S38 S39 S40 L143 L144 | L189 L190 L191 L182 L183 L184 L185 L15 | L15 L185 L186 L187 S123 S124 L188 L189 | L175 L176 L177 S121 S122 L178 L179 L15 | L15 L179 L180 L181 L172 L173 L174 L175 | S47 S48 S49 L149 L150 S50 S51 S52 S53 S54 L18 | L18 S54 S44 S45 S46 S47 | S134 S135 L206 L207 L202 L203 S127 S128 L19 | L19 S128 S129 S130 S131 L204 L205 S132 S133 S134 | L195 L196 L197 S125 S126 L198 L199 L19 | L19 L199 L200 L201 L192 L193 L194 L195
